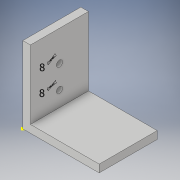
# Autodesk Inventor part: Part1
Saved by Autodesk Inventor 2019 (Build 230136000, 136)
## iProperties
Created: 2020-01-23
Part Number: Part1
Material: Generic
Document SubType Name: Modeling
Designer: pengj5
Density: 1 g/cm^3
Appearance: Default
Author: pengj5
Autodesk Inventor part; units mm, degrees
ref_plane "YZ Plane" through (0, 0, 0) normal (1, 0, 0) x (0, 1, 0)
ref_plane "XZ Plane" through (0, 0, 0) normal (0, 1, 0) x (-1, 0, 0)
ref_plane "XY Plane" through (0, 0, 0) normal (0, 0, 1) x (1, 0, 0)
sketch "Sketch1" plane through (0, 0, 0) normal (0, 1, 0) x (-1, 0, 0)
  line L0 (0, 0) -> (-100, 0)
  line L1 (-100, 0) -> (-100, -76)
  line L2 (-100, -76) -> (0, -76)
  line L3 (0, -76) -> (0, 0)
  dimension "d0" = 100
  dimension "d1" = 76
  constraints: 8 end point, 2 parallel, 1 horizontal, 1 perpendicular
  measures "d0" distance of L2.end L1.end
  measures "d1" distance of L1.end L0.end
extrude "Extrusion1" add sketch "Sketch1" along normal blind 10
sketch "Sketch2" plane through (0, 10, 0) normal (0, 1, 0) x (1, 0, 0)
  line L0 (0, 0) -> (100, 0) projected
  line L1 (100, 76) -> (0, 76) projected
  line L2 (0, 0) -> (10, 0)
  line L3 (10, 0) -> (10, 76)
  line L4 (10, 76) -> (0, 76)
  line L5 (0, 76) -> (0, 0)
  dimension "d4" = 10
  constraints: 8 end point, 2 parallel, 1 horizontal, 1 perpendicular, 1 point on line
  measures "d4" distance of L4.end L3.end
extrude "Extrusion2" add sketch "Sketch2" along normal blind 90
sketch "Sketch3" plane through (10, 10, 0) normal (1, 0, 0) x (0, 0, -1)
  line L0 (0, -10) -> (76, -10) projected
  line L1 (0, -10) -> (38, -10)
  line L2 (38, -10) -> (38, 20)
  circle A0 centre (38, 20) radius 4
  line L3 (38, 20) -> (38, 50)
  circle A1 centre (38, 50) radius 4
  dimension "d7" = 30
  dimension "d8" = 8
  dimension "d9" = 30
  dimension "d10" = 8
  constraints: 6 end point, 2 centre point, 2 coincident, 2 vertical, 1 midpoint
  measures "d7" distance of L1.end L2.end
  measures "d8" diameter of A0
  measures "d9" distance of L3.start L3.end
  measures "d10" diameter of A1
sketch "Sketch4" plane through (0, 0, -76) normal (-1, 0, 0) x (0, 0, 1)
  circle A0 centre (38, 30) radius 4
  circle A1 centre (38, 60) radius 4
  point P0 (76, 0)
  dimension "d15" = 8
  dimension "d16" = 8
  constraints: 2 centre point
  measures "d15" diameter of A0
  measures "d16" diameter of A1
extrude "Extrusion3" cut sketch "Sketch3" against normal blind 10
body "Solid1"
